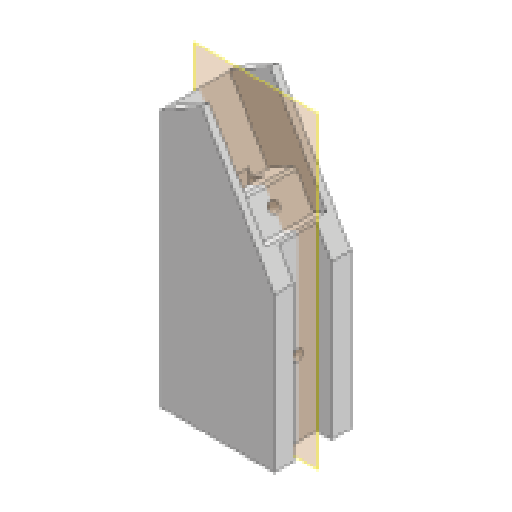
# Autodesk Inventor part: PALM 3
Saved by Autodesk Inventor 2025.1 (Build 291241020, 241B)
## iProperties
Created: 2024-12-04
Part Number: PALM 3
Material: Generic
Document SubType Name: Modeling
Designer: ALEXANDERNICHOLS
Density: 1 g/cm^3
Appearance: Default
Author: ALEXANDERNICHOLS
Autodesk Inventor part; units mm, degrees
ref_plane "YZ Plane" through (0, 0, 0) normal (1, 0, 0) x (0, 1, 0)
ref_plane "XZ Plane" through (0, 0, 0) normal (0, 1, 0) x (-1, 0, 0)
sketch "Sketch1" plane through (0, 0, 0) normal (0, 0, 1) x (1, 0, 0)
  line L0 (0, 0) -> (38.1, 0)
  line L1 (38.1, 0) -> (38.1, 51.7633)
  line L2 (0, 86.36) -> (0, 0)
  line L3 (0, 86.36) -> (13.5942, 94.2086)
  line L4 (0, 86.36) -> (12.7, 64.363)
  line L5 (12.7, 64.363) -> (26.2942, 72.2116)
  line L6 (26.2942, 72.2116) -> (13.5942, 94.2086)
  line L7 (26.2942, 72.2116) -> (38.1, 51.7633)
  dimension "d0" = 15.6972
  dimension "d1" = 25.4
  dimension "d2" = 38.1
  dimension "d3" = 86.36
  dimension "d4" = 120
  constraints: 16 end point, 4 perpendicular, 2 point on line, 1 collinear, 1 horizontal, 1 parallel
  measures "d0" distance between parallel lines of L4 L6
  measures "d1" distance between parallel lines of L5 L3
  measures "d2" distance of L0.start L0.end
  measures "d3" distance from line of L2.start L0
  measures "d4" angle of L2 L3
extrude "Extrusion1" add sketch "Sketch1" along normal blind 20.574 contours L2 L4 L5 L7 L1 L0
sketch "Sketch2" plane through (0, 0, 20.574) normal (0, 0, 1) x (1, 0, 0)
  line L0 (0, 86.36) -> (0, 0) projected
  line L1 (0, 0) -> (38.1, 0) projected
  line L2 (38.1, 0) -> (38.1, 51.7633) projected
  line L3 (38.1, 51.7633) -> (26.2942, 72.2116) projected
  line L4 (26.2942, 72.2116) -> (12.7, 64.363) projected
  line L5 (12.7, 64.363) -> (0, 86.36) projected
  line L6 (26.2942, 72.2116) -> (13.5942, 94.2086)
  line L7 (13.5942, 94.2086) -> (0, 86.36)
  line L8 (38.1, 51.7633) -> (26.2942, 72.2116) projected
  constraints: 4 end point, 1 collinear, 1 perpendicular
extrude "Extrusion2" add sketch "Sketch2" along normal blind 2.54
ref_plane "Work Plane1" through (0, 0, 10.287) normal (0, 0, -1) x (-1, 0, 0)
mirror "Mirror1" about plane through (0, 0, 10.287) normal (0, 0, -1) of "Extrusion2"
sketch "Sketch3" plane through (0, 0, 23.114) normal (0, -1, 0) x (1, 0, 0)
  line L0 (38.1, -25.654) -> (38.1, 0) projected
  line L1 (38.1, -6.477) -> (33.02, -6.477)
  line L2 (33.02, -6.477) -> (33.02, -19.177)
  line L3 (33.02, -19.177) -> (38.1, -19.177)
  line L4 (38.1, -19.177) -> (38.1, -6.477)
  point P0 (0, -23.114)
  point P1 (38.1, -12.827)
  dimension "d9" = 12.7
  dimension "d10" = 6.35
  dimension "d11" = 5.08
  constraints: 8 end point, 2 parallel, 1 horizontal, 1 midpoint, 1 perpendicular, 1 point on line
  measures "d9" distance between parallel lines of L3 L1
  measures "d10" distance from line of point (38.1, -12.827) L3
  measures "d11" distance between parallel lines of L0 L2
extrude "Extrusion3" cut sketch "Sketch3" against normal blind 76.2
sketch "Sketch4" plane through (33.02, 0, 16.637) normal (1, 0, 0) x (0, 0, -1)
  circle A0 centre (6.35, 25.202) radius 1.778 projected
  point P0 (16.637, 0)
extrude "Extrusion4" cut sketch "Sketch4" against normal blind 15.24
sketch "Sketch5" plane through (13.5942, 94.2086, 23.114) normal (0.8660254, 0.5, 0) x (0, 0, -1)
  line L0 (23.114, -25.4) -> (2.54, -25.4) projected
  line L1 (23.114, -25.4) -> (2.54, -25.4)
  line L2 (2.54, -25.4) -> (2.54, -37.7698)
  line L3 (2.54, -37.7698) -> (23.114, -37.7698)
  line L4 (23.114, -37.7698) -> (23.114, -25.4)
  point P0 (23.114, -74.79)
  dimension "d16" = 12.3698
  constraints: 8 end point, 2 parallel, 1 horizontal, 1 perpendicular
  measures "d16" distance between parallel lines of L0 L3
extrude "Extrusion5" cut sketch "Sketch5" against normal blind 5.08
chamfer "Chamfer1" distance 1.016 angle 45 1 edges at (21.893, 69.6706, 10.287)
sketch "Sketch6" plane through (9.1948, 91.6686, 23.114) normal (0.8660254, 0.5, 0) x (0, 0, -1)
  line L0 (22.86, -25.4) -> (2.54, -25.4) projected
  line L1 (23.114, -37.7698) -> (2.54, -37.7698) projected
  circle A0 centre (12.827, -31.5849) radius 1.778
  line L2 (2.54, -37.7698) -> (2.54, 0) projected
  line L3 (2.54, -25.4) -> (2.54, -37.7698)
  point P0 (23.114, -74.79)
  point P1 (12.827, -37.7698)
  point P2 (2.54, -31.5849)
  dimension "d22" = 3.556
  constraints: 2 end point, 2 midpoint, 1 centre point, 1 horizontal alignment, 1 vertical, 1 vertical alignment
  measures "d22" diameter of A0
extrude "Extrusion6" cut sketch "Sketch6" against normal blind 7.62
ref_plane "Work Plane2" through (0, 0, 10.287) normal (0, 0, 1) x (1, 0, 0)
sketch "Sketch7" plane through (0, 0, 10.287) normal (0, 0, 1) x (1, 0, 0)
  line L0 (12.7, 64.363) -> (0, 86.36) projected
  line L1 (21.0149, 69.1636) -> (12.7, 64.363) projected
  line L2 (0, 0) -> (38.1, 0) projected
  line L3 (16.8574, 0) -> (11.3142, 0)
  line L4 (16.51, 66.5627) -> (11.43, 66.5627)
  line L5 (11.43, 66.5627) -> (11.43, 0)
  line L6 (11.43, 0) -> (16.51, 0)
  line L7 (16.51, 0) -> (16.51, 66.5627)
  dimension "d26" = 5.08
  constraints: 10 end point, 5 point on line, 2 parallel, 1 collinear, 1 horizontal, 1 perpendicular
  measures "d26" distance between parallel lines of L7 L5
extrude "Extrusion7" cut sketch "Sketch7" along normal mid plane 10.16 contours L1 L7 L2 L5 L0
sketch "Sketch8" plane through (0, 0, 23.114) normal (-1, 0, 0) x (0, 0, 1)
  circle A0 centre (-12.827, 57.15) radius 1.778 projected
  circle A1 centre (-12.827, 19.05) radius 1.778 projected
  point P0 (-23.114, 0)
extrude "Extrusion8" cut sketch "Sketch8" against normal blind 15.24
sketch "Sketch9" plane through (0, 0, 23.114) normal (0, -1, 0) x (1, 0, 0)
  circle A0 centre (5.08, -12.827) radius 1.778 projected
  circle A1 centre (22.86, -12.827) radius 1.778 projected
  point P0 (0, -23.114)
extrude "Extrusion9" cut sketch "Sketch9" against normal blind 15.24
equation "\"d10\" = 0.5 * d9"
body "Solid1"
